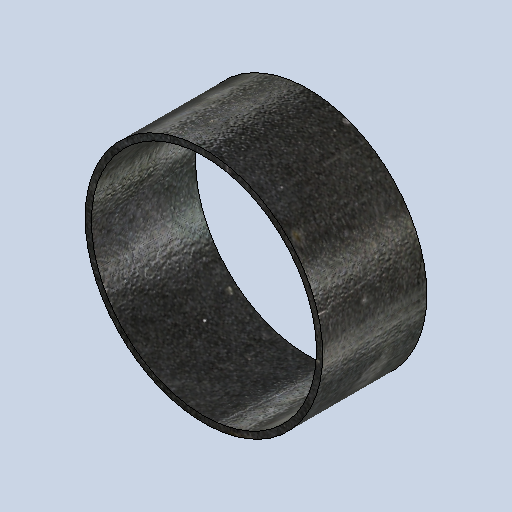
# Autodesk Inventor part: TZS 1442 FDS  tube 1
Saved by Autodesk Inventor 2025 (Build 290162010, 162A)
## iProperties
Created: 2025-02-12
Part Number: TZS 1442 FDS  tube 1
Material: Steel
Document SubType Name: Modeling
Designer: pokla
Density: 7.85 g/cm^3
Appearance: Plate
Mass: 1287.33 g
Surface Area: 1109.67 cm^2
Volume: 163.991 cm^3
Author: pokla
Autodesk Inventor part; units mm, degrees
ref_plane "YZ Plane" through (0, 0, 0) normal (1, 0, 0) x (0, 1, 0)
ref_plane "XZ Plane" through (0, 0, 0) normal (0, 1, 0) x (-1, 0, 0)
ref_plane "XY Plane" through (0, 0, 0) normal (0, 0, 1) x (1, 0, 0)
sketch "Sketch1" plane through (0, 0, 0) normal (0, 1, 0) x (-1, 0, 0)
  circle A0 centre (0, 0) radius 57
  circle A1 centre (0, 0) radius 54
  dimension "d0" = 114
  dimension "d1" = 3
  constraints: 2 centre point, 2 coincident
  measures "d0" diameter of A0
  measures "d1" radial gap between concentric circles of A0 A1
extrude "Extrusion1" add sketch "Sketch1" against normal blind 50
body "Solid1"
